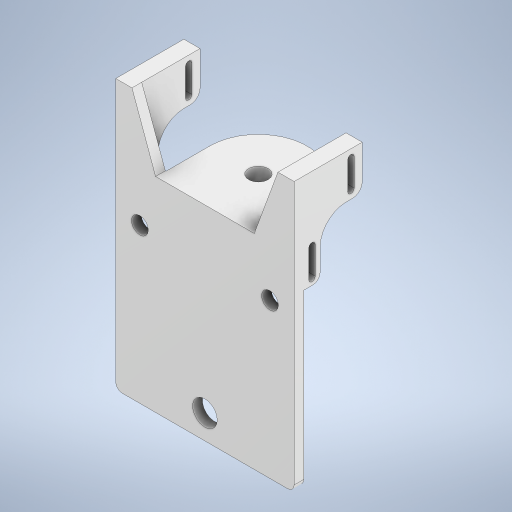
# Autodesk Inventor part: Electromagnet Gantry Plate
Saved by Autodesk Inventor 2023.2 (Build 272271030, 271C)
## iProperties
Created: 2023-04-10
Part Number: Electromagnet Gantry Plate
Material: PC/ABS Plastic
Document SubType Name: Modeling
Designer: ethan
Density: 0.357273 g/cm^3
Appearance: Smooth - White
Author: ethan
Autodesk Inventor part; units mm, degrees
ref_plane "YZ Plane" through (0, 0, 0) normal (1, 0, 0) x (0, 1, 0)
ref_plane "XZ Plane" through (0, 0, 0) normal (0, 1, 0) x (-1, 0, 0)
ref_plane "XY Plane" through (0, 0, 0) normal (0, 0, 1) x (1, 0, 0)
sketch "Sketch1" plane through (0, 0, 0) normal (0, 1, 0) x (-1, 0, 0)
  line L0 (0, 0) -> (55, 0)
  line L1 (55, 0) -> (55, -55)
  line L2 (55, -55) -> (0, -55)
  line L3 (0, -55) -> (0, 0)
  line L4 (47.55, -7.45) -> (7.45, -7.45) construction
  line L5 (7.45, -7.45) -> (7.45, -47.55) construction
  line L6 (7.45, -47.55) -> (47.55, -47.55) construction
  line L7 (47.55, -47.55) -> (47.55, -7.45) construction
  circle A0 centre (47.55, -7.45) radius 2.6
  circle A1 centre (47.55, -47.55) radius 2.6
  circle A2 centre (7.45, -47.55) radius 2.6
  circle A3 centre (7.45, -7.45) radius 2.6
  circle A4 centre (47.55, -7.45) radius 12.5 construction
  circle A5 centre (27.5, -7.45) radius 3.8
  dimension "d0" = 55
  dimension "d1" = 55
  dimension "d2" = 40.1
  dimension "d3" = 40.1
  dimension "d4" = 5.2
  dimension "d5" = 5.2
  dimension "d6" = 5.2
  dimension "d7" = 5.2
  dimension "d8" = 7.45
  dimension "d9" = 7.45
  dimension "d13" = 25
  dimension "d78" = 7.6
  constraints: 16 end point, 6 centre point, 5 coincident, 4 parallel, 2 horizontal, 2 perpendicular, 1 midpoint
  measures "d0" distance of L1.end L2.end
  measures "d1" distance of L0.end L1.end
  measures "d2" distance of L6.end L5.end
  measures "d3" distance of L5.end L4.end
  measures "d4" diameter of A0
  measures "d5" diameter of A3
  measures "d6" diameter of A1
  measures "d7" diameter of A2
  measures "d8" distance between parallel lines of L1 L7
  measures "d9" distance from line of L2 L5.end
  measures "d13" diameter of A4
  measures "d78" diameter of A5
extrude "Extrusion1" add sketch "Sketch1" along normal blind 3 contours L0 L1 L2 L3 | A0 | A3
fillet "Fillet1" radius 2 2 edges at (-55, 1.5, 0) (0, 1.5, 0)
sketch "Sketch3" plane through (0, 0, -53) normal (1, 0, 0) x (0, 0, -1)
  line L0 (-13, 0) -> (-13, -20) construction
  line L1 (12, -20) -> (-13, -20) construction
  line L2 (-13, 0) -> (-33, 0) construction
  line L3 (-33, 0) -> (-33, -20) construction
  line L4 (-33, -20) -> (-13, -20) construction
  line L5 (-13, -20) -> (-13, 0) construction
  line L6 (2, 0) -> (-13, 0) construction
  line L7 (-13, 0) -> (-33, -20) construction
  line L8 (-33, -10) -> (-13, -10) projected
  circle A0 centre (-23, -10) radius 5
  point P0 (-53, 0)
  point P1 (2, -20)
  dimension "d25" = 10
  constraints: 10 end point, 2 parallel, 1 centre point, 1 horizontal, 1 midpoint, 1 perpendicular
  measures "d25" diameter of A0
extrude "Extrusion3" cut sketch "Sketch3" against normal blind 12
sketch "Sketch4" plane through (-55, 0, -2) normal (-1, 0, 0) x (0, 0, 1)
  circle A0 centre (-28, -10) radius 5 projected
  circle A1 centre (-28, -10) radius 2.75
  point P0 (2, 0)
  dimension "d30" = 5.5
  constraints: 1 centre point, 1 coincident
  measures "d30" diameter of A1
extrude "Extrusion4" cut sketch "Sketch4" against normal blind 12 contours A0 | A1
extrude "Extrusion5" cut sketch "Sketch4" against normal through all contours A1
sketch "Sketch5" plane through (-53, 3, 0) normal (0, 0, 1) x (1, 0, 0)
  line L0 (35.5, -3) -> (35.5, -23) construction
  line L1 (15.5, -3) -> (15.5, -23) construction
  line L2 (35.5, -3) -> (15.5, -3) construction
  line L3 (15.5, -3) -> (15.5, -23) construction
  line L4 (15.5, -23) -> (35.5, -23) construction
  line L5 (35.5, -23) -> (35.5, -3) construction
  line L6 (15.5, -23) -> (35.5, -23) construction
  line L7 (15.5, -3) -> (-2, -3) construction
  line L8 (35.5, -23) -> (15.5, -3) construction
  circle A0 centre (25.5, -13) radius 5
  circle A1 centre (25.5, -13) radius 2.75
  point P0 (53, -3)
  dimension "d33" = 10
  dimension "d34" = 5.5
  constraints: 10 end point, 2 centre point, 2 parallel, 1 coincident, 1 horizontal, 1 midpoint, 1 perpendicular
  measures "d33" diameter of A0
  measures "d34" diameter of A1
extrude "Extrusion6" cut sketch "Sketch5" against normal blind 12 contours A0 | A1
ref_plane "Work Plane1" through (0, 0, 0) normal (0, 1, 0) x (1, 0, 0)
sketch "Sketch7" plane through (0, 0, 0) normal (0, 1, 0) x (1, 0, 0)
  line L0 (-19.45, 63) -> (-19.45, 53.4092)
  line L1 (-35.55, 19.45) -> (-35.55, 63) projected
  line L2 (-19.45, 55) -> (-35.55, 55)
  line L3 (-35.55, 55) -> (-35.55, 63)
  line L4 (-35.55, 63) -> (-19.45, 63)
  line L5 (-19.45, 63) -> (-19.45, 55)
  circle A0 centre (-47.55, 47.55) radius 2.6 projected
  circle A1 centre (-47.55, 47.55) radius 12
  circle A2 centre (-7.45, 47.55) radius 2.6 projected
  circle A3 centre (-7.45, 47.55) radius 12
  point P0 (0, 0)
  point P1 (-53, 55)
  dimension "d67" = 24
  dimension "d68" = 24
  constraints: 10 end point, 2 centre point, 2 coincident, 2 parallel, 1 horizontal, 1 perpendicular, 1 point on line
  measures "d67" diameter of A1
  measures "d68" diameter of A3
extrude "Extrusion9" add sketch "Sketch7" along normal blind 25 contours L0 L2 L1 L4
ref_plane "Work Plane3" through (-19.45, -5, -63) normal (0, 0, -1) x (-1, 0, 0)
ref_plane "Work Plane2" through (-19.45, -5, -63) normal (0, 0, -1) x (-1, 0, 0)
sketch "Sketch9" plane through (-19.45, -5, -63) normal (0, 0, -1) x (-1, 0, 0)
  line L0 (0, 0) -> (0, 8) projected
  line L1 (16.1, 8) -> (16.1, 5) projected
  line L2 (0, 8) -> (16.1, 8)
  line L3 (4.55, 8) -> (11.55, 8) projected
  line L4 (8.05, 8) -> (8.05, 21.475)
  circle A0 centre (8.05, 21.475) radius 3
  point P0 (-19.45, 5)
  dimension "d54" = 13.475
  dimension "d55" = 6
  constraints: 4 end point, 1 centre point, 1 coincident, 1 midpoint, 1 perpendicular, 1 vertical
  measures "d54" distance of L4.start L4.end
  measures "d55" diameter of A0
extrude "Extrusion11" cut sketch "Sketch9" against normal through all
sketch "Sketch10" plane through (-19.45, 0, -63) normal (0, 0, -1) x (-1, 0, 0)
  circle A0 centre (8.05, 16.475) radius 3 projected
  arc A1 (23.05, 16.475) -> (-6.95, 16.475) centre (8.05, 16.475) ccw
  line L0 (-6.95, 16.475) -> (-6.95, 0)
  line L1 (23.05, 16.475) -> (23.05, 0)
  line L2 (-6.95, 0) -> (23.05, 0)
  line L3 (33.55, 0) -> (-17.45, 0) projected
  point P0 (-19.45, 0)
  dimension "d60" = 30
  constraints: 6 end point, 2 point on circle, 2 tangent, 2 vertical, 1 centre point, 1 coincident, 1 collinear
  measures "d60" diameter of A1
extrude "Extrusion12" add sketch "Sketch10" against normal up to surface (8 mm away)
chamfer "Chamfer2" distance 6.75 angle 45 1 edges at (-27.5, 31.475, -55)
sketch "Sketch11" plane through (0, 0, 0) normal (0, -1, 0) x (1, 0, 0)
  line L0 (0, -2) -> (0, -55) projected
  line L1 (-19.45, -63) -> (0, -63)
  line L2 (0, -63) -> (0, -55)
  line L3 (0, -55) -> (-19.45, -55)
  line L4 (-19.45, -55) -> (-19.45, -63)
  line L5 (-19.45, -63) -> (-35.55, -63) projected
  line L6 (-55, -55) -> (-55, -2) projected
  line L7 (-35.55, -63) -> (-55, -63)
  line L8 (-55, -63) -> (-55, -55)
  line L9 (-55, -55) -> (-35.55, -55)
  line L10 (-35.55, -55) -> (-35.55, -63)
  point P0 (0, 0)
  constraints: 16 end point, 4 parallel, 2 horizontal, 2 perpendicular
extrude "Extrusion13" add sketch "Sketch11" against normal up to surface (3 mm away)
sketch "Sketch13" plane through (0, 0, 0) normal (0, -1, 0) x (1, 0, 0)
  line L0 (0, -2) -> (0, -63) projected
  line L1 (0, -63) -> (-55, -63)
  line L2 (-55, -63) -> (-55, -83)
  line L3 (-55, -83) -> (0, -83)
  line L4 (0, -83) -> (0, -63)
  point P0 (0, 0)
  dimension "d79" = 20
  constraints: 8 end point, 2 parallel, 1 horizontal, 1 perpendicular
  measures "d79" distance of L2.end L1.end
extrude "Extrusion15" add sketch "Sketch13" against normal up to surface (3 mm away)
sketch "Sketch14" plane through (0, 3, 0) normal (0, 1, 0) x (1, 0, 0)
  line L0 (0, 2) -> (0, 83) projected
  line L1 (0, 80.6806) -> (0, 63)
  line L2 (0, 63) -> (-55, 63)
  line L3 (0, 63) -> (0, 95)
  line L4 (0, 95) -> (-55, 95)
  line L5 (-55, 63) -> (-55, 95)
  point P0 (0, 0)
  dimension "d93" = 32
  constraints: 10 end point, 2 point on line, 1 horizontal, 1 perpendicular
  measures "d93" distance of L1.end L3.end
extrude "Extrusion16" add sketch "Sketch14" along normal blind 25 and the other way blind 3
sketch "Sketch17" plane through (0, 28, -95) normal (0, 0, -1) x (-1, 0, 0)
  arc A0 (37.1007, 0) -> (17.8993, 0) centre (27.5, -11.525) ccw projected
  line L0 (44.95, -28) -> (50.15, -28) projected
  line L1 (46.5, -28) -> (8.5, -28)
  line L2 (5, 0) -> (50, 0)
  line L3 (55, -28) -> (0, -28)
  line L4 (50, -25) -> (5, -25)
  line L5 (50, 0) -> (50, -25)
  line L6 (27.75, -25) -> (27.25, -25) projected
  arc A1 (35.75, -11.525) -> (19.25, -11.525) centre (27.5, -11.525) ccw projected
  line L7 (27.5, -25) -> (27.5, -11.525)
  line L8 (5, 0) -> (5, -25)
  point P0 (55, 0)
  point P1 (40.8949, -25)
  point P2 (50, -28)
  point P3 (39.8, -25)
  point P4 (15.2, -25)
  point P5 (35.55, -13.3305)
  point P6 (19.45, -13.3305)
  point P7 (5, -28)
  dimension "d97" = 3
  constraints: 14 end point, 6 point on line, 2 parallel, 2 symmetric about line, 1 collinear, 1 horizontal, 1 midpoint, 1 perpendicular, 1 vertical
  measures "d97" distance between parallel lines of L1 L4
extrude "Extrusion18" cut sketch "Sketch17" against normal up to surface (32 mm away) contours L2 L5 L4 L8
fillet "Fillet9" radius 8 3 edges at (-39.125, 3, -58.375) (-27.5, 3, -55) (-15.875, 3, -58.375)
sketch "Sketch18" plane through (0, 3, 0) normal (0, 1, 0) x (1, 0, 0)
  circle A0 centre (-47.55, 47.55) radius 2.6 projected
  circle A1 centre (-47.55, 47.55) radius 12 construction
  line L0 (-47.55, 37.5) -> (0, 37.5)
  line L1 (0, 63) -> (0, 2) projected
  line L2 (-47.55, 54.5) -> (0, 54.5)
  line L3 (-47.55, 63) -> (0, 63)
  line L4 (-47.55, 72) -> (0, 72)
  line L5 (-47.55, 80.5) -> (0, 80.5)
  point P0 (0, 0)
  dimension "d106" = 24
  dimension "d107" = 10.05
  dimension "d108" = 17
  dimension "d109" = 8.5
  dimension "d110" = 34.5
  dimension "d111" = 8.5
  constraints: 10 end point, 4 parallel, 1 centre point, 1 coincident, 1 horizontal, 1 point on line
  measures "d106" diameter of A1
  measures "d107" distance of A0.centre L0.start
  measures "d108" distance between parallel lines of L0 L2
  measures "d109" distance between parallel lines of L2 L3
  measures "d110" distance between parallel lines of L0 L4
  measures "d111" distance between parallel lines of L4 L5
sketch "Sketch19" plane through (-55, 0, -2) normal (-1, 0, 0) x (0, 0, 1)
  line L0 (-61, 3) -> (-61, 28) projected
  line L1 (-61, 3) -> (-50.5, 3)
  line L2 (-50.5, 3) -> (-50.5, 8)
  line L3 (-50.5, 8) -> (-61, 8)
  line L4 (-61, 8) -> (-61, 3)
  point P0 (2, 0)
  dimension "d113" = 10.5
  dimension "d114" = 5
  constraints: 8 end point, 2 parallel, 1 horizontal, 1 perpendicular
  measures "d113" distance of L3.end L2.end
  measures "d114" distance of L2.end L1.end
extrude "Extrusion20" add sketch "Sketch19" against normal up to surface (5 mm away)
sketch "Sketch20" plane through (-55, 0, -2) normal (-1, 0, 0) x (0, 0, 1)
  line L0 (2, 0) -> (2, 3) projected
  line L1 (0, 3) -> (-50.5, 3) projected
  line L2 (-35.5, 3) -> (-35.5, 12.0214)
  line L3 (-52.5, 3) -> (-52.5, 12.0214)
  line L4 (-61, 3) -> (-61, 12.0214)
  line L5 (-50.5, 3) -> (-50.5, 8) projected
  arc A0 (-64, 16.5) -> (-64, 18.5) centre (-64, 17.5) ccw projected
  line L6 (-63, 17.5) -> (-82.6938, 17.5)
  line L7 (-78.5, 3) -> (-78.5, 8.5043)
  line L8 (-78.5, 14.9287) -> (-78.5, 19.4859)
  line L9 (-70, 3) -> (-70, 8.5043)
  line L10 (-70, 14.9287) -> (-70, 19.4859)
  line L11 (-50.5, 5.5) -> (-61, 5.5)
  line L12 (-70, 5.5) -> (-79.799, 5.5)
  line L13 (-52.5, 5.5) -> (-61, 5.5) construction
  line L14 (-61, 16.475) -> (-61, 3) projected
  line L15 (-52.5, 6.5) -> (-61, 6.5)
  line L16 (-61, 4.5) -> (-52.5, 4.5)
  arc A1 (-52.5, 4.5) -> (-52.5, 6.5) centre (-52.5, 5.5) ccw
  arc A2 (-61, 6.5) -> (-61, 4.5) centre (-61, 5.5) ccw
  line L17 (-78.5, 5.5) -> (-70, 5.5) construction
  line L18 (-78.5, 4.5) -> (-70, 4.5)
  line L19 (-70, 6.5) -> (-78.5, 6.5)
  arc A3 (-78.5, 6.5) -> (-78.5, 4.5) centre (-78.5, 5.5) ccw
  arc A4 (-70, 4.5) -> (-70, 6.5) centre (-70, 5.5) ccw
  line L20 (-78.5, 17.5) -> (-70, 17.5) construction
  line L21 (-78.5, 16.5) -> (-70, 16.5)
  line L22 (-70, 18.5) -> (-78.5, 18.5)
  arc A5 (-78.5, 18.5) -> (-78.5, 16.5) centre (-78.5, 17.5) ccw
  arc A6 (-70, 16.5) -> (-70, 18.5) centre (-70, 17.5) ccw
  point P0 (-56.75, 5.5)
  point P1 (-74.25, 5.5)
  point P2 (-74.25, 17.5)
  dimension "d123" = 17
  dimension "d125" = 8.5
  dimension "d127" = 2
  dimension "d128" = 2
  dimension "d129" = 2
  constraints: 44 end point, 13 point on circle, 12 tangent, 11 parallel, 11 point on line, 8 perpendicular, 6 centre point, 4 midpoint
  measures "d123" distance between parallel lines of L2 L3
  measures "d125" distance between parallel lines of L3 L4
  measures "d127" diameter of A2
  measures "d128" diameter of A4
  measures "d129" diameter of A6
extrude "Extrusion22" cut sketch "Sketch20" against normal up to surface (5 mm away) contours L16 L4 L11 L3 | L3 L11 A1 | L11 L4 L15 L3 | L3 A1 L11 | A2 L4 | A6 L10 L6 | L6 L10 A6 | L10 L21 L8 L6 | L6 L8 L22 L10 | L8 A5 L6 | L6 A5 L8
sketch "Sketch21" plane through (-55, 0, -2) normal (-1, 0, 0) x (0, 0, 1)
  line L0 (-93, 28) -> (-93, 0) projected
  line L1 (-61, 8) -> (-61, 28) projected
  line L2 (-93, 28) -> (-61, 28)
  line L3 (-61, 28) -> (-61, 21)
  line L4 (-61, 21) -> (-93, 21)
  line L5 (-93, 21) -> (-93, 28)
  point P0 (2, 0)
  dimension "d132" = 7
  constraints: 8 end point, 2 parallel, 1 horizontal, 1 perpendicular, 1 point on line
  measures "d132" distance of L2.end L3.end
extrude "Extrusion23" cut sketch "Sketch21" against normal through all
sketch "Sketch22" plane through (-5, 21, -95) normal (0, 1, 0) x (1, 0, 0)
  line L0 (0, 0) -> (5, 0) projected
  line L1 (5, 0) -> (5, -32) projected
  line L2 (0, 0) -> (5, 0)
  line L3 (5, 0) -> (5, -32)
  line L4 (5, -32) -> (0, -32)
  line L5 (0, -32) -> (0, 0)
  point P0 (5, -95)
  constraints: 8 end point, 2 parallel, 1 horizontal, 1 perpendicular
extrude "Extrusion24" cut sketch "Sketch22" against normal up to surface (18 mm away)
sketch "Sketch23" plane through (0, 0, -2) normal (1, 0, 0) x (0, 0, -1)
  line L0 (0, 0) -> (93, 0) projected
  line L1 (93, 0) -> (50.5, 0)
  line L2 (50.5, 0) -> (50.5, 8)
  line L3 (61, 21) -> (93, 21)
  line L4 (93, 21) -> (93, 0)
  line L5 (61, 8) -> (61, 21) projected
  line L6 (61, 21) -> (61, 8)
  line L7 (61, 8) -> (50.5, 8) projected
  line L8 (61, 8) -> (50.5, 8)
  point P0 (-2, 0)
  point P1 (50.5, 0)
  constraints: 12 end point, 2 parallel, 2 perpendicular, 2 point on line, 1 collinear, 1 horizontal
extrude "Extrusion25" add sketch "Sketch23" against normal blind 5
ref_plane "Work Plane8" through (-27.5, 0, -2) normal (1, 0, 0) x (0, 0, -1)
mirror "Mirror4" about plane through (-27.5, 0, -2) normal (1, 0, 0) of "Extrusion22"
sketch "Sketch24" plane through (0, 0, -2) normal (1, 0, 0) x (0, 0, -1)
  line L0 (0, 0) -> (93, 0) projected
  line L1 (93, 21) -> (81, 21)
  line L2 (81, 21) -> (81, 0)
  line L3 (81, 0) -> (93, 0)
  line L4 (93, 0) -> (93, 21)
  point P0 (-2, 0)
  constraints: 8 end point, 2 parallel, 1 horizontal, 1 perpendicular, 1 point on line
extrude "Extrusion26" cut sketch "Sketch24" against normal through all
fillet "Fillet10" radius 2.25 2 edges at (-2.5, 8, -52.5) (-52.5, 8, -52.5)
sketch "Sketch25" plane through (0, 0, -2) normal (1, 0, 0) x (0, 0, -1)
  line L0 (61, 8) -> (61, 21) projected
  line L1 (61, 21) -> (67.5, 21)
  line L2 (67.5, 21) -> (67.5, 8)
  line L3 (67.5, 8) -> (61, 8)
  line L4 (61, 8) -> (61, 21)
  point P0 (-2, 0)
  dimension "d145" = 6.5
  constraints: 8 end point, 2 parallel, 1 horizontal, 1 perpendicular
  measures "d145" distance of L2.end L3.end
extrude "Extrusion27" cut sketch "Sketch25" against normal through all
fillet "Fillet11" radius 8 2 edges at (-2.5, 8, -69.5) (-52.5, 8, -69.5)
fillet "Fillet12" radius 3 2 edges at (-2.5, 21, -69.5) (-52.5, 21, -69.5)
sketch "Sketch26" plane through (0, 3, 0) normal (0, 1, 0) x (1, 0, 0)
  line L0 (-50, 83) -> (-50, 52.5) projected
  line L1 (-5, 54.5) -> (-5, 63) projected
  line L2 (-50, 83) -> (-5, 83)
  line L3 (-5, 83) -> (-5, 63)
  line L4 (-5, 63) -> (-50, 63)
  line L5 (-50, 63) -> (-50, 83)
  point P0 (0, 0)
  constraints: 8 end point, 2 parallel, 1 horizontal, 1 perpendicular
extrude "Extrusion28" cut sketch "Sketch26" against normal through all
chamfer "Chamfer3" distance 20 angle 20 1 edges at (-50, 1.5, -63) measured on face at (-50, 1.5, -63.5)
chamfer "Chamfer4" distance 20 angle 20 1 edges at (-5, 1.5, -63) measured on face at (-5, 1.5, -63.5)
equation "\"d1\" = d0"
equation "\"d3\" = d2"
equation "\"d5\" = d4"
equation "\"d6\" = d4"
equation "\"d7\" = d4"
equation "\"d8\" = -0.5 * d2 + 0.5 * d0"
equation "\"d9\" = -0.5 * d3 + 0.5 * d1"
body "Solid1"
